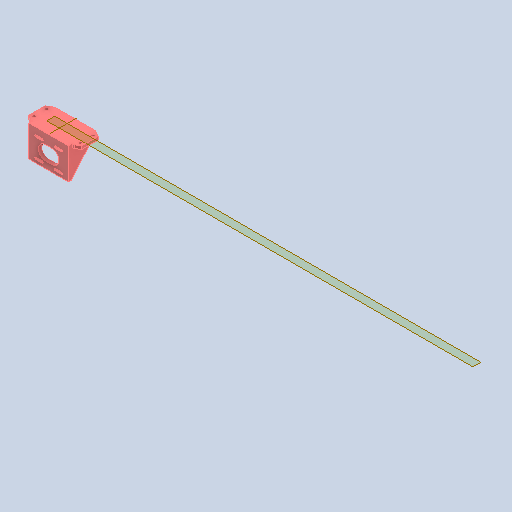
# Autodesk Inventor part: MotorBracketV2
Saved by Autodesk Inventor 2023 (Build 270158000, 158)
## iProperties
Created: 2023-08-18
Part Number: MotorBracketV2
Material: Generic
Document SubType Name: Modeling
Designer: Felix
Density: 1 g/cm^3
Appearance: Smooth - Red
Author: Felix
Autodesk Inventor part; units mm, degrees
ref_plane "XZ Plane" through (0, 0, 0) normal (0, 1, 0) x (-1, 0, 0)
ref_plane "XY Plane" through (0, 0, 0) normal (0, 0, 1) x (1, 0, 0)
ref_plane "Work Plane1" through (-118.9196, 163.4425, 80.2184) normal (0, -1, 0) x (0, 0, -1)
sketch "Sketch1" plane through (-118.9196, 163.4425, 80.2184) normal (0, -1, 0) x (0, 0, -1)
  line L0 (-4.2, -124) -> (-4.2, 744) construction
  line L1 (15.8, -124) -> (15.8, 744) construction
  line L2 (25.8, 100) -> (25.8, 520) construction
  line L3 (-12.85, -53.15) -> (24.8, -53.15)
  line L4 (24.8, -53.15) -> (24.8, 31.85)
  line L5 (24.8, 31.85) -> (-12.85, 31.85)
  line L6 (-12.85, 31.85) -> (-12.85, -53.15)
  line L7 (25.8, -10.65) -> (5.6685, -10.65) construction
  circle A0 centre (15.8, -47.65) radius 5.5 construction
  circle A1 centre (15.8, 26.35) radius 5.5 construction
  line L8 (5.8, -58.8473) -> (5.8, 42.3952) construction
  circle A2 centre (-4.2, -47.65) radius 5.5 construction
  circle A3 centre (-4.2, 26.35) radius 5.5 construction
  point P0 (80.2184, 118.9196)
  point P1 (18.9754, -53.15)
  point P2 (24.8, -26.5615)
  dimension "d0" = 1
  dimension "d1" = 38.65
  dimension "d3" = 11
  dimension "d4" = 63
  dimension "d7" = 0
  dimension "d9" = 10
  dimension "d10" = 10
  constraints: 12 end point, 4 centre point, 3 point on line, 3 symmetric about line, 2 horizontal, 2 parallel, 1 perpendicular, 1 vertical, 4 other
  measures "d0" distance between parallel lines of L2 L4
  measures "d1" distance between parallel lines of L2 L6
  measures "d3" diameter of A0
  measures "d7" distance edge to line of A0 L3
  measures "d9" distance between parallel lines of L1 L8
  measures "d10" distance between parallel lines of L0 L8
extrude "Extrusion1" add sketch "Sketch1" along normal blind 5
ref_plane "Work Plane2" through (-129.5696, 158.4425, 93.0684) normal (1, 0, 0) x (0, 1, 0)
sketch "Sketch4" plane through (-172.0696, 163.4425, 93.0684) normal (0, 0, 1) x (1, 0, 0)
  line L0 (85, 0) -> (0, 0) construction
  line L1 (0, 0) -> (0, -5) construction
  line L2 (85, -5) -> (0, -5) construction
  line L3 (85, 0) -> (85, -5) construction
  line L4 (0, 0) -> (85, 0) construction
  line L5 (42.5, 0) -> (42.5, -58.6666) construction
  line L6 (11, 0) -> (74, 0)
  line L7 (74, 0) -> (74, -50)
  line L8 (74, -50) -> (11, -50)
  line L9 (11, -50) -> (11, 0)
  line L10 (27, -43.5) -> (58, -43.5) construction
  line L11 (58, -43.5) -> (58, -12.5) construction
  line L12 (58, -12.5) -> (27, -12.5) construction
  line L13 (27, -12.5) -> (27, -43.5) construction
  line L14 (27, -43.5) -> (58, -12.5) construction
  line L15 (58, -43.5) -> (27, -12.5) construction
  line L16 (32, -12.5) -> (22, -12.5) construction
  line L17 (32, -10.9) -> (22, -10.9)
  line L18 (22, -14.1) -> (32, -14.1)
  arc A0 (32, -14.1) -> (32, -10.9) centre (32, -12.5) ccw
  arc A1 (22, -10.9) -> (22, -14.1) centre (22, -12.5) ccw
  line L19 (53, -12.5) -> (63, -12.5) construction
  line L20 (53, -14.1) -> (63, -14.1)
  line L21 (63, -10.9) -> (53, -10.9)
  arc A2 (53, -10.9) -> (53, -14.1) centre (53, -12.5) ccw
  arc A3 (63, -14.1) -> (63, -10.9) centre (63, -12.5) ccw
  line L22 (32, -43.5) -> (22, -43.5) construction
  line L23 (32, -45.1) -> (22, -45.1)
  line L24 (22, -41.9) -> (32, -41.9)
  arc A4 (32, -45.1) -> (32, -41.9) centre (32, -43.5) ccw
  arc A5 (22, -41.9) -> (22, -45.1) centre (22, -43.5) ccw
  line L25 (53, -43.5) -> (63, -43.5) construction
  line L26 (53, -45.1) -> (63, -45.1)
  line L27 (63, -41.9) -> (53, -41.9)
  arc A6 (53, -41.9) -> (53, -45.1) centre (53, -43.5) ccw
  arc A7 (63, -45.1) -> (63, -41.9) centre (63, -43.5) ccw
  line L28 (37.5, -28) -> (47.5, -28) construction
  line L29 (37.5, -39.25) -> (47.5, -39.25)
  line L30 (47.5, -16.75) -> (37.5, -16.75)
  arc A8 (37.5, -16.75) -> (37.5, -39.25) centre (37.5, -28) ccw
  arc A9 (47.5, -39.25) -> (47.5, -16.75) centre (47.5, -28) ccw
  point P0 (172.0696, -163.4425)
  point P1 (42.5, -28)
  dimension "d14" = 63
  dimension "d15" = 45
  dimension "d16" = 31
  dimension "d17" = 31
  dimension "d18" = 3.2
  dimension "d19" = 10
  dimension "d21" = 10
  dimension "d22" = 1.6
  dimension "d23" = 10
  dimension "d24" = 10
  dimension "d25" = 1.6
  dimension "d26" = 1.6
  dimension "d27" = 22.5
  dimension "d28" = 10
  constraints: 62 end point, 20 point on circle, 20 tangent, 10 centre point, 9 parallel, 8 midpoint, 4 point on line, 3 horizontal, 3 perpendicular, 1 vertical, 1 other
  measures "d14" distance between parallel lines of L7 L9
  measures "d15" distance between parallel lines of L8 L2
  measures "d16" distance of L12.end L11.end
  measures "d17" distance of L11.end L10.end
  measures "d18" diameter of A1
  measures "d19" distance of L16.start L16.end
  measures "d21" distance of L19.start L19.end
  measures "d22" radius of A3
  measures "d23" distance of L25.start L25.end
  measures "d24" distance of L22.start L22.end
  measures "d25" radius of A5
  measures "d26" radius of A7
  measures "d27" diameter of A9
  measures "d28" distance of L28.start L28.end
extrude "Extrusion2" add sketch "Sketch4" along normal blind 5
sketch "Sketch5" plane through (-161.0696, 113.4425, 93.0684) normal (-1, 0, 0) x (0, 0, 1)
  line L0 (0, 45) -> (0, 0) projected
  line L1 (0, 45) -> (-37.65, 45) projected
  line L2 (-37.65, 50) -> (-37.65, 45) projected
  line L3 (0, 0) -> (0, 45) projected
  line L4 (-37.65, 45) -> (0, 0)
  point P0 (-93.0684, -113.4425)
  constraints: 2 end point
extrude "Extrusion3" add sketch "Sketch5" against normal blind 5
sketch "Sketch6" plane through (-98.0696, 113.4425, 93.0684) normal (1, 0, 0) x (0, 0, -1)
  line L0 (0, 0) -> (37.65, 45) projected
  line L1 (0, 45) -> (37.65, 45) projected
  line L2 (0, 0) -> (0, 45) projected
  point P0 (93.0684, -113.4425)
extrude "Extrusion4" add sketch "Sketch6" against normal blind 5
sketch "Sketch7" plane through (-118.9196, 158.4425, 80.2184) normal (0, -1, 0) x (1, 0, 0)
  circle A0 centre (-47.65, -15.8) radius 5.5 construction
  circle A1 centre (-47.65, 4.2) radius 5.5 construction
  circle A2 centre (26.35, 4.2) radius 5.5 construction
  circle A3 centre (26.35, -15.8) radius 5.5 construction
  point P0 (118.9196, -80.2184)
hole "Hole1" at (-166.5696, 158.4425, 84.4184) at (-166.5696, 158.4425, 64.4184) at (-92.5696, 158.4425, 64.4184) at (-92.5696, 158.4425, 84.4184) direction (0, 1, 0) diameter 5.3 end through all clearance for "Hex Head Cap Screw DIN EN 24017" size "M5" standard "DIN"
sketch "Sketch8" plane through (-118.9196, 158.4425, 80.2184) normal (0, -1, 0) x (1, 0, 0)
  circle A0 centre (-47.65, 4.2) radius 2.65 projected
  circle A1 centre (-47.65, -15.8) radius 2.65 projected
  line L0 (-42.15, -24.8) -> (-42.15, 12.85) projected
  line L1 (-42.15, 12.85) -> (-53.15, 12.85) projected
  line L2 (-53.15, 12.85) -> (-53.15, -24.8) projected
  line L3 (-53.15, -24.8) -> (-42.15, -24.8) projected
  circle A2 centre (26.35, -15.8) radius 2.65 projected
  circle A3 centre (26.35, 4.2) radius 2.65 projected
  line L4 (20.85, 12.85) -> (20.85, -24.8) projected
  line L5 (20.85, -24.8) -> (31.85, -24.8) projected
  line L6 (31.85, -24.8) -> (31.85, 12.85) projected
  line L7 (31.85, 12.85) -> (20.85, 12.85) projected
  line L8 (-53.15, 7.3754) -> (-45.3998, 11.85)
  line L9 (-53.15, -18.9754) -> (-42.15, -25.3263)
  line L10 (31.85, 7.3754) -> (24.0998, 11.85)
  line L11 (31.85, -18.9754) -> (20.85, -25.3263)
  line L12 (-45.3998, 11.85) -> (-42.15, 11.85)
  line L13 (24.0998, 11.85) -> (20.85, 11.85)
  point P0 (118.9196, -80.2184)
  point P1 (37.3678, 12.85)
  point P2 (-28.6678, 12.85)
  point P3 (21.7615, -24.8)
  point P4 (-43.0615, -24.8)
  point P5 (37.3678, 12.85)
  dimension "d42" = 60
  dimension "d43" = 5.5
  dimension "d44" = 60
  dimension "d45" = 5.5
  dimension "d46" = 60
  dimension "d47" = 5.5
  dimension "d48" = 60
  dimension "d49" = 5.5
  dimension "d53" = 7.65
  dimension "d54" = 7.65
  constraints: 12 end point, 8 point on line, 2 perpendicular
  measures "d42" angle of L2 L8
  measures "d43" distance from line of A0.centre L8
  measures "d44" angle of L2 L9
  measures "d45" distance from line of L9 A1.centre
  measures "d46" angle of L6 L10
  measures "d47" distance from line of A3.centre L10
  measures "d48" angle of L6 L11
  measures "d49" distance from line of A2.centre L11
  measures "d53" distance from line of A3.centre L13
  measures "d54" distance from line of A0.centre L12
extrude "Extrusion5" cut sketch "Sketch8" against normal blind 5 contours L12 L8 L2 L1 L0 | L3 L2 L9 | L7 L6 L10 L13 L4 | L11 L6 L5
equation "\"d1\" = MOTOR_HEIGHT"
equation "\"d9\" = d10"
equation "\"d19\" = SLOT_PLAY"
equation "\"d21\" = d19"
equation "\"d22\" = 0.5 * d18"
equation "\"d23\" = d19"
equation "\"d24\" = d19"
equation "\"d25\" = d22"
equation "\"d26\" = d22"
equation "\"d28\" = SLOT_PLAY"
equation "\"d44\" = d42"
equation "\"d45\" = d43"
equation "\"d47\" = d43"
equation "\"d49\" = d45"
equation "\"d54\" = d53"
equation "\"MOTOR_HEIGHT\" = 38.65"
equation "\"SLOT_PLAY\" = 10"
body "Solid1"
